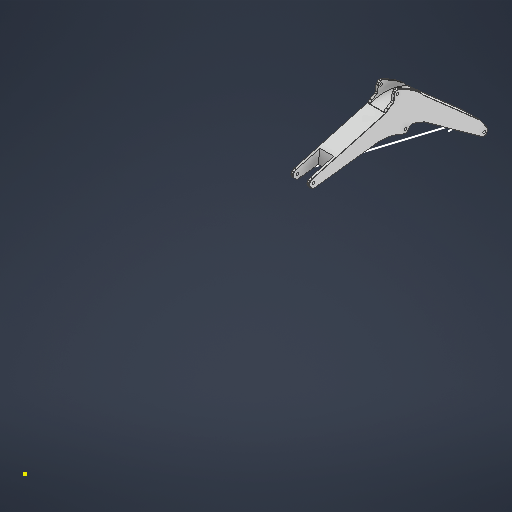
# Autodesk Inventor part: bom
Saved by Autodesk Inventor 2026 (Build 300175000, 175)
## iProperties
Created: 2025-04-29
Part Number: bom
Material: Generic
Document SubType Name: Modeling
Designer: elias
Density: 1 g/cm^3
Appearance: Default
Author: elias
Autodesk Inventor part; units mm, degrees
ref_plane "YZ Plane" through (0, 0, 0) normal (1, 0, 0) x (0, 1, 0)
ref_plane "XZ Plane" through (0, 0, 0) normal (0, 1, 0) x (-1, 0, 0)
ref_plane "XY Plane" through (0, 0, 0) normal (0, 0, 1) x (1, 0, 0)
sketch "Sketch1" plane through (0, 0, 0) normal (1, 0, 0) x (0, 1, 0)
  line L0 (3056.2025, 0) -> (3056.2025, -6694.5386) construction
  line L1 (3056.2025, -6694.5386) -> (0, -6694.5386) construction
  line L2 (0, -6694.5386) -> (0, 0) construction
  line L3 (0, 0) -> (3056.2025, 0) construction
  point P0 (0, 0)
  dimension "d19" = 30
  constraints: 2 end point, 2 other
sketch "Sketch4" plane through (0, 0, 0) normal (1, 0, 0) x (0, 1, 0)
  line L0 (910.8349, -4726.6904) -> (883.9943, -4764.9874)
  line L1 (883.9943, -4764.9874) -> (879.739, -4786.9182)
  line L2 (879.739, -4786.9182) -> (883.9943, -4808.5217)
  line L3 (883.9943, -4808.5217) -> (897.4146, -4817.9274)
  line L4 (897.4146, -4817.9274) -> (926.5466, -4820.96)
  line L5 (926.5466, -4820.96) -> (947.4033, -4816.8519)
  line L6 (947.4033, -4816.8519) -> (969.4262, -4800.3385)
  line L7 (969.4262, -4800.3385) -> (1047.2904, -4749.7016)
  line L8 (1047.2904, -4749.7016) -> (1592.8897, -4130.1299)
  line L9 (1592.8897, -4130.1299) -> (1644.9588, -4082.9591)
  line L10 (1644.9588, -4082.9591) -> (1709.2149, -3998.0333)
  line L11 (1709.2149, -3998.0333) -> (1784.5439, -3864.6138)
  line L12 (1784.5439, -3864.6138) -> (1784.5439, -3825.9608)
  line L13 (1784.5439, -3825.9608) -> (1758.3855, -3811.1918)
  line L14 (1758.3855, -3811.1918) -> (1709.2149, -3806.0731)
  line L15 (1709.2149, -3806.0731) -> (1688.1945, -3803.8848)
  line L16 (1688.1945, -3803.8848) -> (1653.3349, -3744.7771)
  line L17 (1653.3349, -3744.7771) -> (1630.7122, -3719.8052)
  line L18 (1630.7122, -3719.8052) -> (1411.563, -2924.141)
  line L19 (1411.563, -2924.141) -> (1397.6356, -2900.5258)
  line L20 (1397.6356, -2900.5258) -> (1381.6238, -2889.3038)
  line L21 (1381.6238, -2889.3038) -> (1363.2275, -2887.3888)
  line L22 (1363.2275, -2887.3888) -> (1348.6836, -2895.9662)
  line L23 (1348.6836, -2895.9662) -> (1334.2926, -2904.4535)
  line L24 (1334.2926, -2904.4535) -> (1320.4945, -2924.141)
  line L25 (1320.4945, -2924.141) -> (1312.875, -2937.6363)
  line L26 (1312.875, -2937.6363) -> (1316.6848, -2972.5783)
  line L27 (1316.6848, -2972.5783) -> (1397.6356, -3635.1429)
  line L28 (1397.6356, -3635.1429) -> (1395.7611, -3697.8466)
  line L29 (1395.7611, -3697.8466) -> (1390.6708, -3746.7452)
  line L30 (1390.6708, -3746.7452) -> (1381.6238, -3793.3718)
  line L31 (1381.6238, -3793.3718) -> (1365.4628, -3841.0444)
  line L32 (1365.4628, -3841.0444) -> (1352.8702, -3871.0567)
  line L33 (1352.8702, -3871.0567) -> (1338.8616, -3889.5715)
  line L34 (1338.8616, -3889.5715) -> (1336.8025, -3909.3513)
  line L35 (1336.8025, -3909.3513) -> (1333.3216, -3942.7892)
  line L36 (1333.3216, -3942.7892) -> (1359.1665, -3971.3179)
  line L37 (1359.1665, -3971.3179) -> (1381.6238, -3980.7405)
  line L38 (1381.6238, -3980.7405) -> (1386.3469, -4012.7674)
  line L39 (1386.3469, -4012.7674) -> (1372.4257, -4045.9462)
  line L40 (1372.4257, -4045.9462) -> (1349.2863, -4101.0951)
  line L41 (1341.4881, -4130.1299) -> (908.605, -4729.8721)
  circle A0 centre (1364.2337, -2936.1395) radius 15
  circle A1 centre (1748.9253, -3843.5008) radius 15
  circle A2 centre (1375.6214, -3932.1004) radius 15
  circle A3 centre (920.5041, -4786.9182) radius 15
  line L42 (1349.2863, -4101.0951) -> (1341.4881, -4130.1299)
  point P0 (0, 0)
  dimension "d17" = 30
  dimension "d19" = 30
  dimension "d20" = 30
  dimension "d21" = 30
  constraints: 86 end point, 10 point on line, 9 parallel, 9 perpendicular, 4 centre point, 1 vertical
  measures "d17" diameter of A0
  measures "d19" diameter of A1
  measures "d20" diameter of A2
  measures "d21" diameter of A3
extrude "Extrusion1" add sketch "Sketch4" along normal mid plane 200
fillet "Fillet1" radius 20 32 edges at (0, 1381.6238, -2889.3038) (0, 1363.2275, -2887.3888) (0, 1334.2926, -2904.4535) (0, 1320.4945, -2924.141) (0, 1312.875, -2937.6363) (0, 1316.6848, -2972.5783) (0, 1397.6356, -2900.5258) (0, 1411.563, -2924.141) (0, 1653.3349, -3744.7771) (0, 1630.7122, -3719.8052) (0, 1688.1945, -3803.8848) (0, 1758.3855, -3811.1918) (0, 1784.5439, -3825.9608) (0, 1784.5439, -3864.6138) (0, 1709.2149, -3998.0333) (0, 1644.9588, -4082.9591) (0, 1592.8897, -4130.1299) (0, 1047.2904, -4749.7016) (0, 969.4262, -4800.3385) (0, 947.4033, -4816.8519) (0, 926.5466, -4820.96) (0, 897.4146, -4817.9274) (0, 883.9943, -4808.5217) (0, 879.739, -4786.9182) (0, 883.9943, -4764.9874) (0, 1341.4881, -4130.1299) (0, 1386.3469, -4012.7674) (0, 1381.6238, -3980.7405) (0, 1359.1665, -3971.3179) (0, 1333.3216, -3942.7892) (0, 1338.8616, -3889.5715) (0, 1352.8702, -3871.0567)
fillet "Fillet2" radius 2 142 edges at (100, 1339.5717, -3889.8516) (100, 1336.2651, -3914.5139) (100, 1335.13, -3942.1976) (100, 1347.7492, -3958.7149) (100, 1359.4485, -3970.9195) (100, 1367.2438, -3974.7069) (100, 1379.2838, -3982.5565) (100, 1384.4016, -3999.5763) (100, 1385.5904, -4012.672) (100, 1366.7381, -4059.5016) (100, 1345.863, -4113.8411) (100, 1341.1868, -4129.9867) (100, 1123.9731, -4431.4883) (100, 897.5219, -4745.6858) (100, 884.4071, -4765.1627) (100, 881.8334, -4776.1242) (100, 880.1177, -4786.9177) (100, 881.467, -4795.6907) (100, 885.3, -4807.6718) (100, 891.875, -4814.0449) (100, 897.6462, -4817.3074) (100, 913.0663, -4819.5567) (100, 926.5364, -4820.7359) (100, 936.2088, -4819.0568) (100, 947.194, -4816.3818) (100, 959.974, -4807.426) (100, 969.4325, -4800.3477) (100, 1007.4903, -4775.5846) (100, 1047.1683, -4749.5604) (100, 1320.6222, -4439.3114) (100, 1592.9124, -4130.1522) (100, 1618.6475, -4106.7953) (100, 1644.8941, -4082.8999) (100, 1677.2486, -4040.2825) (100, 1709.1775, -3998.0087) (100, 1745.9166, -3933.0289) (100, 1783.887, -3864.4412) (100, 1784.5439, -3848.4971) (100, 1781.8161, -3827.5532) (100, 1768.1929, -3816.7291) (100, 1758.2553, -3811.5998) (100, 1726.2368, -3807.8451) (100, 1689.491, -3801.8657) (100, 1668.7207, -3770.8652) (100, 1653.2514, -3744.8386) (100, 1642.937, -3733.2994) (100, 1631.2018, -3719.5362) (100, 1520.8583, -3320.959) (100, 1411.4013, -2924.2095) (100, 1405.025, -2913.0552) (100, 1397.295, -2900.8406) (100, 1389.9799, -2895.1602) (100, 1381.3922, -2889.9238) (100, 1373.1231, -2888.4189) (100, 1363.4528, -2888.4222) (100, 1347.7877, -2896.4946) (100, 1334.6074, -2904.7941) (100, 1326.4298, -2915.6724) (100, 1320.5145, -2924.1537) (100, 1318.0273, -2928.5109) (100, 1313.8641, -2937.8396) (100, 1315.1216, -2958.2414) (100, 1316.6852, -2972.5783) (100, 1357.1681, -3303.925) (100, 1396.6984, -3666.4948) (100, 1393.216, -3722.2959) (100, 1386.1473, -3770.0585) (100, 1373.5433, -3817.2081) (100, 1359.6535, -3854.8898) (100, 1352.7334, -3870.9779) (100, 1346.7892, -3879.0938) (-100, 1339.5717, -3889.8516) (-100, 1346.7892, -3879.0938) (-100, 1352.7334, -3870.9779) (-100, 1359.6535, -3854.8898) (-100, 1373.5433, -3817.2081) (-100, 1386.1473, -3770.0585) (-100, 1393.216, -3722.2959) (-100, 1396.6984, -3666.4948) (-100, 1357.1681, -3303.925) (-100, 1316.6852, -2972.5783) (-100, 1315.1216, -2958.2414) (-100, 1313.8641, -2937.8396) (-100, 1318.0273, -2928.5109) (-100, 1320.5145, -2924.1537) (-100, 1326.4298, -2915.6724) (-100, 1334.6074, -2904.7941) (-100, 1347.7877, -2896.4946) (-100, 1363.4528, -2888.4222) (-100, 1373.1231, -2888.4189) (-100, 1381.3922, -2889.9238) (-100, 1389.9799, -2895.1602) (-100, 1397.295, -2900.8406) (-100, 1405.025, -2913.0552) (-100, 1411.4013, -2924.2095) (-100, 1520.8583, -3320.959) (-100, 1631.2018, -3719.5362) (-100, 1642.937, -3733.2994) (-100, 1653.2514, -3744.8386) (-100, 1668.7207, -3770.8652) (-100, 1689.491, -3801.8657) (-100, 1726.2368, -3807.8451) (-100, 1758.2553, -3811.5998) (-100, 1768.1929, -3816.7291) (-100, 1781.8161, -3827.5532) (-100, 1784.5439, -3848.4971) (-100, 1783.887, -3864.4412) (-100, 1745.9166, -3933.0289) (-100, 1709.1775, -3998.0087) (-100, 1677.2486, -4040.2825) (-100, 1644.8941, -4082.8999) (-100, 1618.6475, -4106.7953) (-100, 1592.9124, -4130.1522) (-100, 1320.6222, -4439.3114) (-100, 1047.1683, -4749.5604) (-100, 1007.4903, -4775.5846) (-100, 969.4325, -4800.3477) (-100, 959.974, -4807.426) (-100, 947.194, -4816.3818) (-100, 936.2088, -4819.0568) (-100, 926.5364, -4820.7359) (-100, 913.0663, -4819.5567) (-100, 897.6462, -4817.3074) (-100, 891.875, -4814.0449) (-100, 885.3, -4807.6718) (-100, 881.467, -4795.6907) (-100, 880.1177, -4786.9177) (-100, 881.8334, -4776.1242) (-100, 884.4071, -4765.1627) (-100, 897.5219, -4745.6858) (-100, 1123.9731, -4431.4883) (-100, 1341.1868, -4129.9867) (-100, 1345.863, -4113.8411) (-100, 1366.7381, -4059.5016) (-100, 1385.5904, -4012.672) (-100, 1384.4016, -3999.5763) (-100, 1379.2838, -3982.5565) (-100, 1367.2438, -3974.7069) (-100, 1359.4485, -3970.9195) (-100, 1347.7492, -3958.7149) (-100, 1335.13, -3942.1976) (-100, 1336.2651, -3914.5139)
sketch "Sketch6" plane through (0, 0, 0) normal (1, 0, 0) x (0, 1, 0)
  arc A0 (1629.4482, -3715.216) -> (1633.9081, -3723.333) centre (1648.7302, -3709.9052) ccw projected
  line L0 (1631.998, -3715.216) -> (1629.4482, -3715.216)
  line L1 (1631.998, -3715.216) -> (1794.3064, -3709.9052)
  line L2 (1794.3064, -3709.9052) -> (1794.3064, -4169.5412)
  line L3 (1794.3064, -4169.5412) -> (1588.1369, -4169.5412)
  line L4 (1049.1005, -4747.6461) -> (1592.144, -4130.9768) projected
  line L5 (1588.1369, -4169.5412) -> (1592.144, -4130.9768)
  arc A1 (1592.144, -4130.9768) -> (1629.4482, -3715.216) centre (1163.2686, -3882.9418) ccw
  point P0 (0, 0)
  constraints: 10 end point, 2 point on circle, 1 centre point, 1 horizontal, 1 perpendicular, 1 vertical
extrude "Extrusion2" cut sketch "Sketch6" along normal mid plane 150 contours L0 L1 L2 L3 L5 A1
sketch "Sketch7" plane through (0, 0, 0) normal (1, 0, 0) x (0, 1, 0)
  line L0 (1327.8786, -3157.0345) -> (1514.0487, -3184.5541)
  line L1 (1514.0487, -3184.5541) -> (1514.0487, -2822.2026)
  line L2 (1514.0487, -2822.2026) -> (1269.0991, -2822.2026)
  line L3 (1269.0991, -2822.2026) -> (1327.8786, -3157.0345)
  point P0 (0, 0)
  constraints: 8 end point, 1 perpendicular, 1 vertical
extrude "Extrusion3" cut sketch "Sketch7" along normal mid plane 150
sketch "Sketch8" plane through (0, 0, 0) normal (1, 0, 0) x (0, 1, 0)
  line L0 (1316.7005, -2972.7071) -> (1397.6356, -3635.1429) projected
  line L1 (1397.6356, -3635.1429) -> (1426.2154, -3869.0623)
  arc A0 (1339.3411, -4133.1044) -> (1426.2154, -3869.0623) centre (1101.9373, -3908.682) ccw
  line L2 (1397.6356, -3635.1429) -> (1203.7021, -3635.1429)
  line L3 (1203.7021, -3635.1429) -> (1203.7021, -4133.1044)
  line L4 (1203.7021, -4133.1044) -> (1339.3411, -4133.1044)
  point P0 (0, 0)
  constraints: 8 end point, 2 perpendicular, 2 point on circle, 1 centre point, 1 collinear, 1 horizontal, 1 tangent
extrude "Extrusion4" cut sketch "Sketch8" along normal mid plane 150
sketch "Sketch9" plane through (-100, 0, 0) normal (-1, 0, 0) x (0, 0, 1)
  circle A0 centre (-2936.1395, 1364.2337) radius 15 projected
  circle A1 centre (-4786.9182, 920.5041) radius 15 projected
  line L0 (-2936.1395, 1364.2337) -> (-4786.9182, 920.5041)
  line L1 (-4786.9182, 920.5041) -> (-4599.6104, 920.5041)
  point P0 (0, 0)
  constraints: 4 end point, 1 horizontal
body "Solid1"
